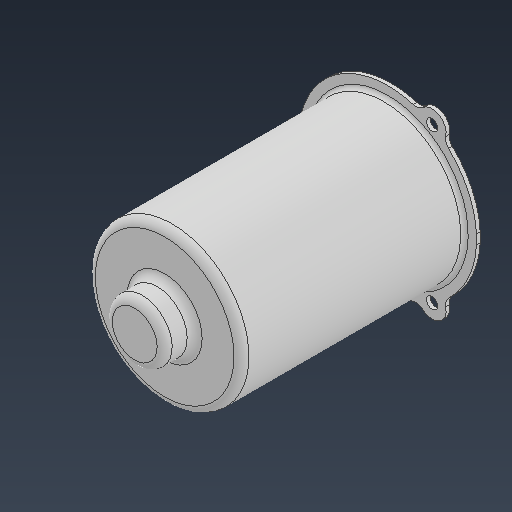
# Autodesk Inventor part: MCEN4000:M3
Saved by Autodesk Inventor 2021 (Build 250183000, 183)
## iProperties
Created: 2020-10-18
Part Number: MCEN4000:M3
Material: Generic
Document SubType Name: Modeling
Designer: Eugene Tang
Mass: 77.3779 g
Surface Area: 762.148 cm^2
Volume: 77.3779 cm^3
Density: 1 g/cm^3
Appearance: Default
Description: MOTOR COVER
Author: Eugene Tang
Autodesk Inventor part; units mm, degrees
ref_plane "YZ Plane" through (0, 0, 0) normal (1, 0, 0) x (0, 1, 0)
ref_plane "XZ Plane" through (0, 0, 0) normal (0, 1, 0) x (-1, 0, 0)
ref_plane "XY Plane" through (0, 0, 0) normal (0, 0, 1) x (1, 0, 0)
sketch "Sketch2" plane through (0, 0, 0) normal (0, 0, 1) x (1, 0, 0)
  arc A0 (34.8026, 39.4269) -> (22.3684, 46.6058) centre (27.5, 41.1362) ccw construction
  circle A1 centre (3.75, 0) radius 7.5 construction
  circle A2 centre (3.75, 0) radius 55 construction
  point P0 (0, 0)
  dimension "d0" = 110
  constraints: 1 centre point, 1 coincident, 1 tangent
  measures "d0" diameter of A2
ref_plane "Work Plane1" through (3.75, 10, 0) normal (-1, 0, 0) x (0, 1, 0)
sketch "Sketch3" plane through (3.75, 10, 0) normal (-1, 0, 0) x (0, 1, 0)
  line L0 (25, 0) -> (25, -115) construction
  line L1 (-45, -115) -> (25, -115) construction
  line L2 (0, -115) -> (0, -135) construction
  line L3 (-20, -135) -> (0, -135) construction
  line L4 (-65, 0) -> (45, 0) construction
  line L5 (45, 0) -> (25, 0) construction
  line L6 (25, 0) -> (25, -115) construction
  line L7 (25, -115) -> (0, -115) construction
  line L8 (0, -115) -> (0, -135) construction
  line L9 (0, -135) -> (-10, -135) construction
  line L10 (-10, -135) -> (-10, 0) construction
  line L11 (-10, 0) -> (25, 0) construction
  line L12 (-14, 4) -> (-14, -139) construction
  line L13 (-14, -139) -> (4, -139) construction
  line L14 (4, -139) -> (4, -119) construction
  line L15 (4, -119) -> (29, -119) construction
  line L16 (29, -119) -> (29, 4) construction
  line L17 (29, 4) -> (-14, 4) construction
  line L18 (31, 6) -> (31, -121) construction
  line L19 (31, -121) -> (6, -121) construction
  line L20 (6, -121) -> (6, -141) construction
  line L21 (6, -141) -> (-16, -141) construction
  line L22 (-16, -141) -> (-16, 6) construction
  line L23 (-16, 6) -> (31, 6) construction
  line L24 (45, 0) -> (31, 0)
  line L25 (4, -131) -> (4, -123)
  line L26 (8, -119) -> (25, -119)
  line L27 (29, -115) -> (29, -2)
  line L28 (33, -2) -> (45, -2)
  line L29 (31, -4) -> (31, -117)
  line L30 (27, -121) -> (10, -121)
  line L31 (6, -125) -> (6, -133)
  line L32 (45, 0) -> (45, -2)
  arc A0 (33, -2) -> (31, -4) centre (33, -4) ccw
  arc A1 (31, 0) -> (29, -2) centre (31, -2) ccw
  arc A2 (25, -119) -> (29, -115) centre (25, -115) ccw
  arc A3 (10, -121) -> (6, -125) centre (10, -125) ccw
  arc A4 (0, -135) -> (4, -131) centre (0, -131) ccw
  arc A5 (2, -137) -> (6, -133) centre (2, -133) ccw
  arc A6 (8, -119) -> (4, -123) centre (8, -123) ccw
  arc A7 (27, -121) -> (31, -117) centre (27, -117) ccw
  line L33 (-10, -135) -> (-10, -137)
  line L34 (2, -137) -> (-10, -137)
  line L35 (-10, -135) -> (0, -135)
  line L36 (-10, -170.4) -> (-10, 35.4) projected
  point P0 (-16, 0)
  point P1 (29, 0)
  point P2 (31, -2)
  dimension "d1" = 4
  dimension "d2" = 2
  dimension "d3" = 2
  dimension "d4" = 2
  dimension "d5" = 4
  dimension "d7" = 4
  dimension "d8" = 4
  dimension "d9" = 2
  constraints: 66 end point, 18 point on line, 16 point on circle, 16 tangent, 9 perpendicular, 8 centre point, 7 collinear, 4 equal radius, 2 vertical, 1 horizontal, 1 midpoint, 1 parallel, 14 other
  measures "d1" distance between parallel lines of L10 L12
  measures "d2" distance between parallel lines of L16 L18
  measures "d3" distance between parallel lines of L4 L28
  measures "d4" radius of A0
  measures "d5" radius of A2
  measures "d7" radius of A4
  measures "d8" radius of A5
  measures "d9" distance between parallel lines of L3 L34
revolve "Revolution1" add sketch "Sketch3" angle 360 about axis through (3.75, 0, -40) along (0, 0, -1)
ref_plane "Work Plane2" through (0, 0, -25) normal (0, 0, -1) x (-1, 0, 0)
sketch "Sketch4" plane through (0, 0, -25) normal (0, 0, -1) x (-1, 0, 0)
  circle A0 centre (-3.75, 0) radius 55 projected
  arc A1 (-34.8026, -39.4269) -> (-22.3684, -46.6058) centre (-27.5, -41.1362) ccw projected
  arc A2 (-17.5, -45.4663) -> (-22.3684, -46.6058) centre (-18.9474, -50.2523) ccw projected
  arc A3 (-17.5, -45.4663) -> (42.5, -10.8253) centre (-3.75, 0) ccw projected
  arc A4 (45.9211, -7.1789) -> (42.5, -10.8253) centre (47.3684, -11.9648) ccw projected
  arc A5 (45.9211, -7.1789) -> (45.9211, 7.1789) centre (43.75, 0) ccw projected
  arc A6 (42.5, 10.8253) -> (45.9211, 7.1789) centre (47.3684, 11.9648) ccw projected
  arc A7 (42.5, 10.8253) -> (-17.5, 45.4663) centre (-3.75, 0) ccw projected
  arc A8 (-22.3684, 46.6058) -> (-17.5, 45.4663) centre (-18.9474, 50.2523) ccw projected
  arc A9 (-22.3684, 46.6058) -> (-34.8026, 39.4269) centre (-27.5, 41.1362) ccw projected
  arc A10 (-36.25, 34.641) -> (-34.8026, 39.4269) centre (-39.6711, 38.2874) ccw projected
  arc A11 (-36.25, 34.641) -> (-51.1842, 2.5) centre (-3.75, 0) ccw projected
  line L0 (-51.1842, 2.5) -> (-51.25, 2.5) projected
  line L1 (-51.25, 2.5) -> (-51.25, -2.5) projected
  line L2 (-51.25, -2.5) -> (-51.1842, -2.5) projected
  arc A12 (-51.1842, -2.5) -> (-36.25, -34.641) centre (-3.75, 0) ccw projected
  arc A13 (-34.8026, -39.4269) -> (-36.25, -34.641) centre (-39.6711, -38.2874) ccw projected
  circle A14 centre (-3.75, 0) radius 10 projected
  circle A15 centre (-27.5, -41.1362) radius 3 projected
  circle A16 centre (-27.5, -41.1362) radius 3 projected
  circle A17 centre (-27.5, 41.1362) radius 3 projected
  circle A18 centre (43.75, 0) radius 3 projected
  arc A19 (-17.5, -45.4663) -> (-22.3684, -46.6058) centre (-18.9474, -50.2523) ccw projected
  arc A20 (-17.5, -45.4663) -> (42.5, -10.8253) centre (-3.75, 0) ccw projected
  arc A21 (45.9211, -7.1789) -> (42.5, -10.8253) centre (47.3684, -11.9648) ccw projected
  arc A22 (45.9211, -7.1789) -> (45.9211, 7.1789) centre (43.75, 0) ccw projected
  arc A23 (42.5, 10.8253) -> (45.9211, 7.1789) centre (47.3684, 11.9648) ccw projected
  arc A24 (42.5, 10.8253) -> (-17.5, 45.4663) centre (-3.75, 0) ccw projected
  arc A25 (-22.3684, 46.6058) -> (-17.5, 45.4663) centre (-18.9474, 50.2523) ccw projected
  arc A26 (-22.3684, 46.6058) -> (-34.8026, 39.4269) centre (-27.5, 41.1362) ccw projected
  arc A27 (-36.25, 34.641) -> (-34.8026, 39.4269) centre (-39.6711, 38.2874) ccw projected
  arc A28 (-36.25, 34.641) -> (-51.1842, 2.5) centre (-3.75, 0) ccw projected
  line L3 (-51.1842, 2.5) -> (-51.25, 2.5) projected
  line L4 (-51.25, 2.5) -> (-51.25, -2.5) projected
  line L5 (-51.25, -2.5) -> (-51.1842, -2.5) projected
  arc A29 (-51.1842, -2.5) -> (-36.25, -34.641) centre (-3.75, 0) ccw projected
  arc A30 (-34.8026, -39.4269) -> (-36.25, -34.641) centre (-39.6711, -38.2874) ccw projected
  arc A31 (-34.8026, -39.4269) -> (-22.3684, -46.6058) centre (-27.5, -41.1362) ccw projected
  circle A32 centre (-3.75, 0) radius 10 projected
  point P0 (0, 0)
  point P1 (-31.25, 47.6314)
  point P2 (-31.25, -47.6314)
  point P3 (51.25, 0)
extrude "Extrusion1" cut sketch "Sketch4" against normal up to surface (146 mm away) contours A5 A6 A7 A8 A9 A0 | A0 A1 A2 A3 A4 A5 | A9 A10 A11 L0 L1 L2 A12 A13 A1 A0 | A15 | A17 | A18
equation "\"d3\" = d2"
equation "\"d9\" = d2"
equation "\"d6\" = d2"
body "Solid1"
